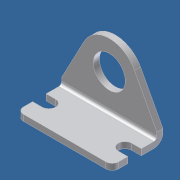
# Autodesk Inventor part: D-129
Saved by Autodesk Inventor 2012 (Build 160160000, 160)
## iProperties
Category: PARTsolutions
Created: 2013-01-19
Part Number: D-129
Catalog Web Link: www.cadenas.de
Description: Mounting Brackets for Original Line Cylinders -
Document SubType Name: Modeling
Designer: PARTsolutions
Material: Default
Density: 1 g/cm^3
NB: D-129
NN: Mounting Brackets for Original Line Cylinders
NBSYN: $PN1.
LINA: D-129
PN: D-129
PSPN: 0.63 (D-129)
PN1: D-129
MAT: Zinc-Plated Carbon Steel
A: 1.38
A1: 1.38000
B: 1.88
B1: 1.87500
C: 1.00
C1: 1.00000
D: 0.63
D1: 0.62900
E: 0.27
E1: 0.26600
F: 0.56
F1: 0.56000
G: 0.81
G1: 0.81000
H: 0.12
H1: 0.12000
I: 0.56
I1: 0.56200
J: 1.50
J1: 1.50000
K: 0.13
K1: 0.12500
L: 0.25
L1: 0.25000
M: 0.06200
N: 0.00000
SHP: 2
ASSCFGPRA: mounting_bracket2
COLOR: 0.75,0.75,0.75,0.00
KT: DUMMY
SUPPLIER: Bimba
ARTICLENO: D-129
BOMINFO: D-129
CREATOR: CADENAS GmbH
PSOL_IDENT_0: {\\10.0.0.242\data_v9\23d-libs\bimba\bimba\bimba_imperial\bimba_full_line\original_line_cylinders\ac
PSOL_IDENT_1: cessories\mounting_bracket.prj},191 {VTYP=3D},{NB=D-129},{LINA=D-129},{NN=Mounting Brackets for Orig
PSOL_IDENT_2: inal Line Cylinders},{DATE=26.09.2012 12:25:43},{GEOMDATE=27.08.2012 00:00:00},{VERSION=},{LINEID=60
PSOL_IDENT_3: },{LINESUBID=-1},{WBVAR=}  {NB=D-129},{LINA=D-129},{KT=DUMMY},{PN=D-129},{PSPN=0.63 (D-129)},{PN1=D-
PSOL_IDENT_4: 129},{MAT=Zinc-Plated Carbon Steel},{A=1.38},{A1=1.38000},{B=1.88},{B1=1.87500},{C=1.00},{C1=1.00000
PSOL_IDENT_5: },{D=0.63},{D1=0.62900},{E=0.27},{E1=0.26600},{F=0.56},{F1=0.56000},{G=0.81},{G1=0.81000},{H=0.12},{
PSOL_IDENT_6: H1=0.12000},{I=0.56},{I1=0.56200},{J=1.50},{J1=1.50000},{K=0.13},{K1=0.12500},{L=0.25},{L1=0.25000},
PSOL_IDENT_7: {M=0.06200},{N=0.00000},{SHP=2},{ASSCFGPRA=mounting_bracket2},{COLOR=0.75,0.75,0.75,0.00}
Title: D-129
Author: Cadenas PARTsolutions
Autodesk Inventor part; units mm, degrees
sketch "Sketch_1" plane through (0, 0, 0) normal (1, 0, 0) x (0, 1, 0)
  line L0 (0, 25.4) -> (0, 4.6228)
  arc A0 (0, 4.6228) -> (4.6228, 0) centre (4.6228, 4.6228) ccw
  line L1 (4.6228, 0) -> (42.0624, 0)
  line L2 (42.0624, 0) -> (42.0624, 3.048)
  line L3 (42.0624, 3.048) -> (4.6228, 3.048)
  arc A1 (3.048, 4.6228) -> (4.6228, 3.048) centre (4.6228, 4.6228) ccw
  line L4 (3.048, 4.6228) -> (3.048, 25.4)
  line L5 (3.048, 25.4) -> (0, 25.4)
  constraints: 12 end point, 4 point on circle, 2 centre point
extrude "Extrusion1" add sketch "Sketch_1" along normal blind 47.625
sketch "Sketch_2" plane through (0, 0, 0) normal (0, 0, 1) x (1, 0, 0)
  line L0 (-9.525, -3.5052) -> (57.15, -3.5052)
  line L1 (57.15, -3.5052) -> (57.15, 56.0832)
  line L2 (57.15, 56.0832) -> (-9.525, 56.0832)
  line L3 (-9.525, 56.0832) -> (-9.525, -3.5052)
  line L4 (-3.3686, 0) -> (50.9936, 0)
  line L5 (50.9936, 0) -> (36.4228, 27.4668)
  arc A0 (36.4228, 27.4668) -> (11.2022, 27.4668) centre (23.8125, 20.7772) ccw
  line L6 (11.2022, 27.4668) -> (-3.3686, 0)
  constraints: 14 end point, 2 point on circle, 1 centre point
extrude "Extrusion2" cut sketch "Sketch_2" along normal blind 4.572
sketch "Sketch_3" plane through (0, 0, 0) normal (0, 0, 1) x (1, 0, 0)
  circle A0 centre (23.8125, 20.574) radius 7.9883
  constraints: 1 centre point
extrude "Extrusion3" cut sketch "Sketch_3" along normal blind 4.572
sketch "Sketch_6" plane through (0, 0, 0) normal (0, 1, 0) x (-1, 0, 0)
  line L0 (23.8125, 22.225) -> (23.8125, 32.512)
  line L1 (23.8125, 32.512) -> (-3.175, 32.512)
  line L2 (-3.175, 32.512) -> (-3.175, 25.4)
  arc A0 (0, 22.225) -> (-3.175, 25.4) centre (-3.175, 22.225) ccw
  line L3 (0, 22.225) -> (23.8125, 22.225)
  constraints: 8 end point, 2 point on circle, 1 centre point
extrude "Extrusion4" cut sketch "Sketch_6" along normal blind 4.572
sketch "Sketch_7" plane through (0, 0, 0) normal (0, 1, 0) x (-1, 0, 0)
  line L0 (-44.45, 32.512) -> (-71.4375, 32.512)
  line L1 (-71.4375, 32.512) -> (-71.4375, 22.225)
  line L2 (-71.4375, 22.225) -> (-47.625, 22.225)
  arc A0 (-44.45, 25.4) -> (-47.625, 22.225) centre (-44.45, 22.225) ccw
  line L3 (-44.45, 25.4) -> (-44.45, 32.512)
  constraints: 8 end point, 2 point on circle, 1 centre point
extrude "Extrusion5" cut sketch "Sketch_7" along normal blind 4.572
sketch "Sketch_8" plane through (0, 0, 0) normal (0, 1, 0) x (-1, 0, 0)
  line L0 (4.7625, 17.6022) -> (-4.7625, 17.6022)
  arc A0 (-4.7625, 17.6022) -> (-4.7625, 10.8458) centre (-4.7625, 14.224) ccw
  line L1 (-4.7625, 10.8458) -> (4.7625, 10.8458)
  line L2 (4.7625, 10.8458) -> (4.7625, 17.6022)
  constraints: 6 end point, 2 point on circle, 1 centre point
extrude "Extrusion6" cut sketch "Sketch_8" along normal blind 4.572
sketch "Sketch_9" plane through (0, 0, 0) normal (0, 1, 0) x (-1, 0, 0)
  arc A0 (-42.8625, 10.8458) -> (-42.8625, 17.6022) centre (-42.8625, 14.224) ccw
  line L0 (-42.8625, 17.6022) -> (-52.3875, 17.6022)
  line L1 (-52.3875, 17.6022) -> (-52.3875, 10.8458)
  line L2 (-52.3875, 10.8458) -> (-42.8625, 10.8458)
  constraints: 6 end point, 2 point on circle, 1 centre point
extrude "Extrusion7" cut sketch "Sketch_9" along normal blind 4.572
ref_plane "h1_XY" through (23.8125, 0, 25.4) normal (1, 0, 0) x (0, 0, -1)
ref_plane "h1_YZ" through (23.8125, 0, 25.4) normal (0, 0, -1) x (0, 1, 0)
ref_plane "h1_ZX" through (23.8125, 0, 25.4) normal (0, 1, 0) x (1, 0, 0)
ref_plane "d1_XY" through (23.8125, 12.5857, 0) normal (1, 0, 0) x (0, 0, -1)
ref_plane "d1_YZ" through (23.8125, 12.5857, 0) normal (0, 0, -1) x (0, 1, 0)
ref_plane "d1_ZX" through (23.8125, 12.5857, 0) normal (0, 1, 0) x (1, 0, 0)
ref_plane "h2_XY" through (23.8125, 3.048, 25.4) normal (1, 0, 0) x (0, 0, -1)
ref_plane "h2_YZ" through (23.8125, 3.048, 25.4) normal (0, 0, -1) x (0, 1, 0)
ref_plane "h2_ZX" through (23.8125, 3.048, 25.4) normal (0, 1, 0) x (1, 0, 0)
ref_plane "d2_XY" through (23.8125, 28.5623, 0) normal (1, 0, 0) x (0, 0, -1)
ref_plane "d2_YZ" through (23.8125, 28.5623, 0) normal (0, 0, -1) x (0, 1, 0)
ref_plane "d2_ZX" through (23.8125, 28.5623, 0) normal (0, 1, 0) x (1, 0, 0)
ref_plane "h3_XY" through (23.8125, 20.574, 3.048) normal (1, 0, 0) x (0, 0, -1)
ref_plane "h3_YZ" through (23.8125, 20.574, 3.048) normal (0, 0, -1) x (0, 1, 0)
ref_plane "h3_ZX" through (23.8125, 20.574, 3.048) normal (0, 1, 0) x (1, 0, 0)
ref_plane "h4_XY" through (23.8125, 35.052, 3.048) normal (1, 0, 0) x (0, 0, -1)
ref_plane "h4_YZ" through (23.8125, 35.052, 3.048) normal (0, 0, -1) x (0, 1, 0)
ref_plane "h4_ZX" through (23.8125, 35.052, 3.048) normal (0, 1, 0) x (1, 0, 0)
ref_plane "h5_XY" through (47.625, 6.35, 0) normal (1, 0, 0) x (0, 0, -1)
ref_plane "h5_YZ" through (47.625, 6.35, 0) normal (0, 0, -1) x (0, 1, 0)
ref_plane "h5_ZX" through (47.625, 6.35, 0) normal (0, 1, 0) x (1, 0, 0)
ref_plane "h6_XY" through (47.625, 0, 0) normal (1, 0, 0) x (0, 0, -1)
ref_plane "h6_YZ" through (47.625, 0, 0) normal (0, 0, -1) x (0, 1, 0)
ref_plane "h6_ZX" through (47.625, 0, 0) normal (0, 1, 0) x (1, 0, 0)
ref_plane "l1_XY" through (0, 0, 0) normal (0, 1, 0) x (1, 0, 0)
ref_plane "l1_YZ" through (0, 0, 0) normal (1, 0, 0) x (0, 0, -1)
ref_plane "l1_ZX" through (0, 0, 0) normal (0, 0, -1) x (0, 1, 0)
ref_plane "l2_XY" through (47.625, 0, 0) normal (0, 1, 0) x (1, 0, 0)
ref_plane "l2_YZ" through (47.625, 0, 0) normal (1, 0, 0) x (0, 0, -1)
ref_plane "l2_ZX" through (47.625, 0, 0) normal (0, 0, -1) x (0, 1, 0)
ref_plane "l3_XY" through (0, 0, 25.4) normal (0, 1, 0) x (1, 0, 0)
ref_plane "l3_YZ" through (0, 0, 25.4) normal (1, 0, 0) x (0, 0, -1)
ref_plane "l3_ZX" through (0, 0, 25.4) normal (0, 0, -1) x (0, 1, 0)
ref_plane "l4_XY" through (0, 0, 14.224) normal (0, 1, 0) x (1, 0, 0)
ref_plane "l4_YZ" through (0, 0, 14.224) normal (1, 0, 0) x (0, 0, -1)
ref_plane "l4_ZX" through (0, 0, 14.224) normal (0, 0, -1) x (0, 1, 0)
ref_plane "l5_XY" through (4.7625, 0, 14.224) normal (0, 1, 0) x (1, 0, 0)
ref_plane "l5_YZ" through (4.7625, 0, 14.224) normal (1, 0, 0) x (0, 0, -1)
ref_plane "l5_ZX" through (4.7625, 0, 14.224) normal (0, 0, -1) x (0, 1, 0)
ref_plane "l6_XY" through (42.8625, 0, 14.224) normal (0, 1, 0) x (1, 0, 0)
ref_plane "l6_YZ" through (42.8625, 0, 14.224) normal (1, 0, 0) x (0, 0, -1)
ref_plane "l6_ZX" through (42.8625, 0, 14.224) normal (0, 0, -1) x (0, 1, 0)
ref_plane "l7_XY" through (42.8625, 0, 17.6022) normal (0, 1, 0) x (1, 0, 0)
ref_plane "l7_YZ" through (42.8625, 0, 17.6022) normal (1, 0, 0) x (0, 0, -1)
ref_plane "l7_ZX" through (42.8625, 0, 17.6022) normal (0, 0, -1) x (0, 1, 0)
ref_plane "l8_XY" through (42.8625, 0, 10.8458) normal (0, 1, 0) x (1, 0, 0)
ref_plane "l8_YZ" through (42.8625, 0, 10.8458) normal (1, 0, 0) x (0, 0, -1)
ref_plane "l8_ZX" through (42.8625, 0, 10.8458) normal (0, 0, -1) x (0, 1, 0)
ref_plane "mounting_bracket_XY" through (23.8125, 20.574, 3.048) normal (0, 0, 1) x (1, 0, 0)
ref_plane "mounting_bracket_YZ" through (23.8125, 20.574, 3.048) normal (1, 0, 0) x (0, 1, 0)
ref_plane "mounting_bracket_ZX" through (23.8125, 20.574, 3.048) normal (0, 1, 0) x (0, 0, 1)
ref_plane "mounting_bracket_1_XY" through (23.8125, 20.574, 0) normal (0, 0, 1) x (1, 0, 0)
ref_plane "mounting_bracket_1_YZ" through (23.8125, 20.574, 0) normal (1, 0, 0) x (0, 1, 0)
ref_plane "mounting_bracket_1_ZX" through (23.8125, 20.574, 0) normal (0, 1, 0) x (0, 0, 1)
body "Solid1"
